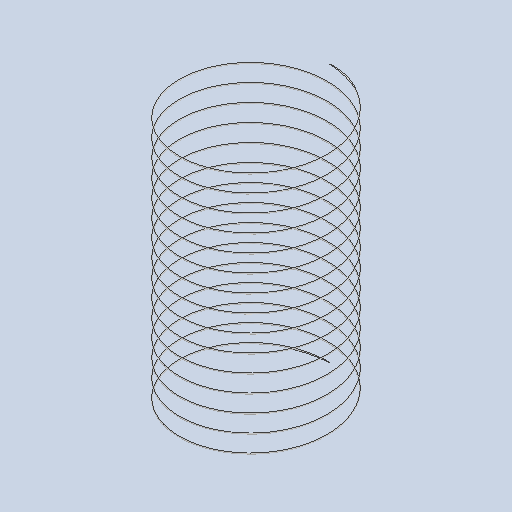
# Autodesk Inventor part: Spring
Saved by Autodesk Inventor 2023 (Build 270158000, 158)
## iProperties
Created: 2025-06-02
Part Number: Spring
Material: Generic
Document SubType Name: Modeling
Designer: dylan
Density: 1 g/cm^3
Appearance: Default
Author: dylan
Autodesk Inventor part; units mm, degrees
ref_plane "YZ Plane" through (0, 0, 0) normal (1, 0, 0) x (0, 1, 0)
ref_plane "XZ Plane" through (0, 0, 0) normal (0, 1, 0) x (-1, 0, 0)
ref_plane "XY Plane" through (0, 0, 0) normal (0, 0, 1) x (1, 0, 0)
sketch "Sketch1" plane through (0, 0, 0) normal (0, 1, 0) x (-1, 0, 0)
  circle A0 centre (0, 0) radius 600
  dimension "d0" = 1200
  constraints: 1 centre point, 1 coincident
  measures "d0" diameter of A0
extrude "Extrusion1" add sketch "Sketch1" along normal blind 2000
sketch "Sketch2" plane through (0, 0, 0) normal (1, 0, 0) x (0, 1, 0)
  circle A0 centre (-5, -570) radius 5
  line L0 (0, -600) -> (0, 600) projected
  line L1 (0, -600) -> (2000, -600) projected
  point P0 (0, 0)
  dimension "d3" = 10
  dimension "d4" = 30
  constraints: 1 centre point, 1 tangent
  measures "d3" diameter of A0
  measures "d4" distance from line of L1 A0.centre
coil "Coil1" sketch "Sketch2" operation intersect axis through (0, -10, 0) along (0, 1, 0) pitch 134 turns 15 hand right
body "Solid1"
